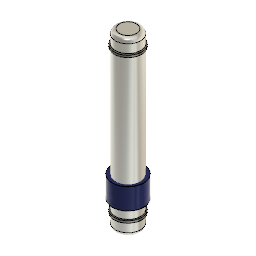
Pino_Rotação_Dribler (Autodesk Fusion 360 design; units mm, degrees)
Autodesk Fusion 360 part; units mm, degrees
sketch "Esboço1" plane through (0, 0, 0) normal (0, 0, 1) x (1, 0, 0)
  circle A0 centre (0, 0) radius 6
  dimension "d1" = 12
  constraint coincident A0.centre origin
  measures "d1" diameter of A0
extrude "Extrusão1" add sketch "Esboço1" along normal blind 81.5 makes body 1
fillet "Arredondamento1" radius 2 2 edges at (-5.594, -2.1697, 81.5) (-5.594, -2.1697, 0) on bodies 1
ref_plane "Plano de trabalho1" through (0, 0, 12) normal (0, 0, 1) x (1, 0, 0)
ref_plane "Plano de trabalho2" through (0, 0, 6) normal (0, 0, 1) x (1, 0, 0)
ref_plane "Plano de trabalho3" through (0, 0, 75.5) normal (0, 0, 1) x (1, 0, 0)
sketch "Esboço2" plane through (0, 0, 75.5) normal (0, 0, 1) x (1, 0, 0)
  circle A0 centre (0, 0) radius 6.25
  circle A1 centre (0, 0) radius 5.25
  dimension "d9" = 12.5
  dimension "d12" = 10.5
  constraint coincident A0.centre A1.centre
  measures "d9" diameter of A0
  measures "d12" diameter of A1
extrude "Extrusão2" cut sketch "Esboço2" against normal blind 1.5 bodies 1
ref_plane "Plano de trabalho4" through (0, 0, 75.2) normal (0, 0, 1) x (1, 0, 0)
sketch "Esboço3" plane through (0, 0, 75.2) normal (0, 0, 1) x (1, 0, 0)
  circle A0 centre (0, 0) radius 5.25
  circle A1 centre (0, 0) radius 6.5
  dimension "d13" = 13
  dimension "d14" = 10.5
  constraint coincident A0.centre A1.centre
  constraint concentric A0 A1
  measures "d13" diameter of A1
  measures "d14" diameter of A0
extrude "Extrusão3" add sketch "Esboço3" against normal blind 1 separate body makes body 2
sketch "Esboço4" plane through (0, 0, 12) normal (0, 0, 1) x (1, 0, 0)
  circle A0 centre (0, 0) radius 7.5
  dimension "d18" = 15
  constraint coincident A0.centre origin
  measures "d18" diameter of A0
extrude "Extrusão4" add sketch "Esboço4" along normal blind 10 separate body makes body 3
sketch "Esboço5" plane through (0, 0, 6) normal (0, 0, 1) x (1, 0, 0)
  circle A0 centre (0, 0) radius 7
  circle A1 centre (0, 0) radius 5.25
  dimension "d21" = 10.5
  dimension "d22" = 14
  constraint coincident A0.centre A1.centre
  measures "d21" diameter of A1
  measures "d22" diameter of A0
extrude "Extrusão5" cut sketch "Esboço5" along normal blind 1.5 bodies 1
ref_plane "Plano de trabalho5" through (0, 0, 6.3) normal (0, 0, 1) x (1, 0, 0)
sketch "Esboço6" plane through (0, 0, 6.3) normal (0, 0, 1) x (1, 0, 0)
  circle A0 centre (0, 0) radius 5.25
  circle A1 centre (0, 0) radius 6.5
  dimension "d26" = 10.5
  dimension "d27" = 13
  constraint coincident A0.centre A1.centre
  measures "d26" diameter of A0
  measures "d27" diameter of A1
extrude "Extrusão6" add sketch "Esboço6" along normal blind 1 separate body makes body 4
